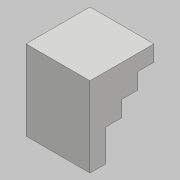
# Autodesk Inventor part: 15
Saved by Autodesk Inventor 2018 (Build 220112000, 112)
## iProperties
Created: 2020-11-05
Part Number: 15
Material: 一般
Document SubType Name: Modeling
Designer: 王鼎鈞
Density: 1 g/cm^3
Appearance: 預設
Author: 王鼎鈞
Autodesk Inventor part; units mm, degrees
ref_plane "YZ Plane" through (0, 0, 0) normal (1, 0, 0) x (0, 1, 0)
ref_plane "XZ Plane" through (0, 0, 0) normal (0, 1, 0) x (-1, 0, 0)
ref_plane "XY Plane" through (0, 0, 0) normal (0, 0, 1) x (1, 0, 0)
sketch "草圖1" plane through (0, 0, 0) normal (1, 0, 0) x (0, 1, 0)
  line L0 (0, -3.5) -> (0, 3.5) projected
  line L1 (-2.8, 0) -> (2.8, 0) projected
  line L2 (-2, -2.5) -> (2, -2.5)
  line L3 (2, -2.5) -> (2, 2.5)
  line L4 (2, 2.5) -> (-2, 2.5)
  line L5 (-2, 2.5) -> (-2, -2.5)
  line L6 (-2, -2.5) -> (2, 2.5) construction
  line L7 (2, -2.5) -> (-2, 2.5) construction
  point P0 (0, 0)
  dimension "d0" = 4
  dimension "d1" = 5
  constraints: 12 end point, 2 midpoint, 2 parallel, 1 horizontal, 1 perpendicular
  measures "d0" distance of L4.end L3.end
  measures "d1" distance of L3.end L2.end
extrude "擠出1" add sketch "草圖1" along normal blind 4
sketch "草圖2" plane through (4, 0, 0) normal (1, 0, 0) x (0, 0, -1)
  line L0 (0, -2.8) -> (0, 2.8) projected
  line L1 (3.5, 0) -> (-3.5, 0) projected
  line L2 (2.5, -2) -> (2.5, 2) projected
  line L3 (2.5, 2) -> (0.5, 2)
  line L4 (2.5, 2) -> (2.5, 0)
  line L5 (2.5, 0) -> (0.5, 2)
  line L6 (2.5, 2) -> (-2.5, 2) projected
  line L7 (-2.5, 2) -> (-1.5, 2)
  line L8 (-1.5, 2) -> (-1.5, 1)
  line L9 (-1.5, 1) -> (-0.5, 1)
  line L10 (-0.5, 1) -> (-0.5, 0)
  line L11 (-0.5, 0) -> (1.5, 0)
  line L12 (1.5, 0) -> (1.5, -1)
  line L13 (1.5, -1) -> (2.5, -1)
  line L14 (2.5, -1) -> (2.5, -2)
  line L15 (-2.5, 2) -> (-2.5, -2) projected
  line L16 (2.5, -2) -> (-2.5, -2)
  line L17 (-2.5, -2) -> (-2.5, 2)
  point P0 (0, 0)
  dimension "d4" = 2
  dimension "d5" = 2
  dimension "d6" = 1
  dimension "d7" = 1
  dimension "d8" = 1
  dimension "d9" = 1
  dimension "d10" = 2
  dimension "d11" = 1
  constraints: 26 end point, 6 perpendicular, 4 point on line, 2 horizontal, 1 midpoint
  measures "d4" distance of L2.end L3.end
  measures "d5" distance of L2.end L4.end
  measures "d6" distance of L6.end L7.end
  measures "d7" distance of L7.end L8.end
  measures "d8" distance of L8.end L9.end
  measures "d9" distance of L9.end L10.end
  measures "d10" distance of L10.end L11.end
  measures "d11" distance of L11.end L12.end
extrude "擠出2" cut sketch "草圖2" against normal blind 1000 contours L3 L2 L5
extrude "擠出3" cut sketch "草圖2" against normal blind 3 contours L1 L10 L9 L8 L6 L0 | L0 L6 L5 L1 | L1 L2 L13 L12
sketch "草圖3" plane through (4, 0, 0.5) normal (0, 1, 0) x (1, 0, 0)
  line L0 (0, 2) -> (0, 0) projected
  line L1 (0, 2) -> (-3, 2) projected
  line L2 (-3, 2) -> (-3, 0) projected
  line L3 (0, 0) -> (-3, 0) projected
  line L4 (0, 2) -> (0, 1)
  line L5 (0, -2) -> (0, 3) projected
  line L6 (0, 1) -> (-3, 2)
  point P0 (-4, 0.5)
  dimension "d16" = 1
  constraints: 4 end point, 1 point on line
  measures "d16" distance of L0.start L4.end
extrude "擠出4" cut sketch "草圖3" against normal blind 1 contours L0 L6 L1
